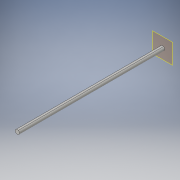
# Autodesk Inventor part: Bucket - Axle
Saved by Autodesk Inventor 2016 (Build 200138000, 138)
## iProperties
Created: 2015-08-29
Part Number: Bucket - Axle
Material: Generic
Description: Axle - 250 mm
Document SubType Name: Modeling
Designer: PTC
Density: 1 g/cm^3
Appearance: Default
Sending System: Creo  TM  2.0  (c) 2012
PROJECT: FTC
PTC_MATERIAL_NAME: METAL_ALUMINIUM_5052
NIKCONFIGCOUNT: 1
Author: phi
Autodesk Inventor part; units mm, degrees
ref_plane "FRONT" through (0, 0, 0) normal (0, 0, 1) x (1, 0, 0)
ref_plane "TOP" through (0, 0, 0) normal (0, 1, 0) x (-1, 0, 0)
ref_plane "RIGHT" through (0, 0, 0) normal (1, 0, 0) x (0, 1, 0)
ref_plane "Work Plane4" through (0, 0, 125) normal (0, 0, 1) x (1, 0, 0)
sketch "Sketch1" plane through (0, 0, 125) normal (0, 0, 1) x (1, 0, 0)
  arc A0 (-1.0878, 2.1) -> (1.0878, 2.1) centre (0, 0) ccw projected
  line L0 (1.0878, 2.1) -> (-1.0878, 2.1) projected
extrude "Extrusion1" add sketch "Sketch1" along normal blind 160
body "Solid2"
